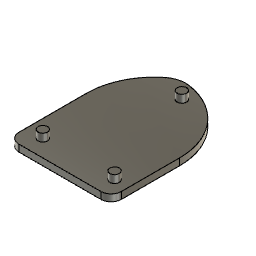
Roboter-Platte-Test (Autodesk Fusion 360 design; units mm, degrees)
Autodesk Fusion 360 part; units mm, degrees
sketch "Skizze1" plane through (0, 0, 0) normal (0, 0, 1) x (1, 0, 0)
sketch "Skizze2" plane through (0, 0, 0) normal (0, 0, 1) x (1, 0, 0)
  circle A0 centre (0, 0) radius 1.4
  circle A1 centre (21, 0) radius 1.4
  circle A2 centre (10.5, 30.2) radius 1.4
  line L0 (-5, -5) -> (25, -5)
  line L1 (25, -5) -> (25, 35)
  line L2 (25, 35) -> (-5, 35)
  line L3 (-5, 35) -> (-5, -5)
  dimension "d1" = 2.8
  dimension "d2" = 2.8
  dimension "d3" = 21
  dimension "d5" = 2.8
  dimension "d6" = 30.2
  dimension "d7" = 10.5
  constraint coincident A0.centre origin
  constraint horizontal L0
  constraint vertical L1
  constraint horizontal L2
  constraint vertical L3
  measures "d1" diameter of A0
  measures "d2" diameter of A1
  measures "d3" distance of A1.centre A0.centre
  measures "d5" diameter of A2
  measures "d6" vertical distance of A0.centre A2.centre
  measures "d7" horizontal distance of A0.centre A2.centre
extrude "Extrusion1" add sketch "Skizze2" along normal blind 2
extrude "Extrusion2" add sketch "Skizze2" along normal blind 4.25 contours A2
extrude "Extrusion3" add sketch "Skizze2" along normal blind 4.25 contours A0 | A1
fillet "Abrundung1" radius 3 1 edges at (25, -5, 1)
fillet "Abrundung2" radius 20 1 edges at (25, 35, 1)
fillet "Abrundung3" radius 20 1 edges at (-5, 35, 1)
fillet "Abrundung4" radius 3 1 edges at (-5, -5, 1)
fillet "Abrundung5" radius 7 1 edges at (5, 35, 1)
equation "d3 = 23.8 mm - 2.8 mm"
equation "d6 = 33 mm - 2.8 mm"
equation "d7 = ( 21 / 2 ) * 1 mm"
